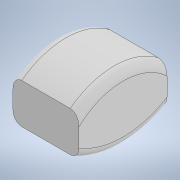
# Autodesk Inventor part: Weapon-Healing-Stock
Saved by Autodesk Inventor 2020 (Build 240168000, 168)
## iProperties
Created: 2019-12-04
Part Number: Weapon-Healing-Stock
Material: Generic
Document SubType Name: Modeling
Designer: vifly_01
Density: 1 g/cm^3
Appearance: Default
Author: vifly_01
Autodesk Inventor part; units mm, degrees
ref_plane "YZ Plane" through (0, 0, 0) normal (1, 0, 0) x (0, 1, 0)
ref_plane "XZ Plane" through (0, 0, 0) normal (0, 1, 0) x (-1, 0, 0)
ref_plane "XY Plane" through (0, 0, 0) normal (0, 0, 1) x (1, 0, 0)
sketch "Sketch1" plane through (0, 0, 0) normal (0, 0, 1) x (1, 0, 0)
  line L0 (7.5, -7.5) -> (-7.5, -7.5)
  line L1 (-7.5, -7.5) -> (-7.5, 7.5)
  line L2 (-7.5, 7.5) -> (7.5, 7.5)
  line L3 (7.5, 7.5) -> (7.5, -7.5)
  line L4 (7.5, -7.5) -> (-7.5, 7.5) construction
  line L5 (-7.5, -7.5) -> (7.5, 7.5) construction
  point P0 (0, 0)
  dimension "d0" = 15
  dimension "d1" = 15
  constraints: 12 end point, 2 midpoint, 2 parallel, 1 horizontal, 1 perpendicular
  measures "d0" distance of L1.end L2.end
  measures "d1" distance of L0.end L1.end
extrude "Extrusion1" add sketch "Sketch1" along normal blind 20
sketch "Sketch2" plane through (7.5, -7.5, 0) normal (1, 0, 0) x (0, 0, -1)
  line L0 (0, 0) -> (0, 15) projected
  line L1 (-20, 0) -> (-20, 15) projected
  arc A0 (0, 11.6201) -> (-20, 11.6201) centre (-10, -1.4833) ccw
  line L2 (0, 15) -> (-20, 15) projected
  line L3 (-20, 11.6201) -> (0, 11.6201) construction
  line L4 (-20, 11.6201) -> (0, 11.6201) construction
  arc A1 (-20, 2.519) -> (0, 2.519) centre (-10, 21.1088) ccw
  line L5 (-20, 2.519) -> (0, 2.519) construction
  line L6 (-20, 2.519) -> (0, 2.519) construction
  line L7 (-20, 11.6201) -> (-20, 15)
  line L8 (-20, 15) -> (-10, 15)
  line L9 (-10, 15) -> (0, 15)
  line L10 (0, 15) -> (0, 11.6201)
  line L11 (0, 2.519) -> (0, 0)
  line L12 (0, 0) -> (-10, 0)
  line L13 (0, 0) -> (-20, 0) projected
  line L14 (-10, 0) -> (-20, 0)
  line L15 (-20, 0) -> (-20, 2.519)
  point P0 (0, 7.5)
  point P1 (-20, 2.519)
  point P2 (0, 2.519)
  point P3 (-10, 15)
  dimension "d4" = 0
  dimension "d5" = 0
  constraints: 24 end point, 6 collinear, 4 point on circle, 3 tangent, 2 centre point, 2 horizontal, 2 midpoint, 2 point on line, 1 perpendicular
  measures "d4" distance between parallel lines of L3 L4
  measures "d5" distance between parallel lines of L5 L6
extrude "Extrusion2" cut sketch "Sketch2" against normal blind 20 contours L12 A1 L0 | L13 L1 A1 | A0 L2 L0 | A0 L1 L2
fillet "Fillet1" radius 2 4 edges at (7.5, 7.5, 10) (7.5, -7.5, 10) (-7.5, -7.5, 10) (-7.5, 7.5, 10)
body "Solid1"
